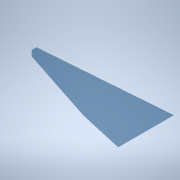
# Autodesk Inventor part: Receivingbeam_OXS200_11728845
Saved by Autodesk Inventor 2021 (Build 250183000, 183)
## iProperties
Created: 2025-06-20
Part Number: Receivingbeam_OXS200_11728845
Material: Generic
Catalog Web Link: www.cadenas.de
Description: ox_receiving_beam-receiving beam
Vendor: BAUMER
Document SubType Name: Modeling
Designer: psAdmin
Manufacturer: BAUMER
Mass: 161.252 g
Surface Area: 402.746 cm^2
Volume: 161.252 cm^3
Density: 1 g/cm^3
Appearance: PSOLRGB-29-191-255
Category: PARTsolutions
Company: BAUMER
Title: Receivingbeam_OXS200_11728845
Author: Cadenas PARTsolutions
Comments: receiving beam
PSOL_IDENT_0: {$CADENAS_DATA/23d-libs/baumer/products/smartvisionsensors/smartprofilesensors/oxmp/oxmp_receiving_b
PSOL_IDENT_1: eam.prj},210 {VTYP=3D},{NB=Receivingbeam_OXS200_11728845},{LINA=Receivingbeam_OXS200_11728845},{NN=o
PSOL_IDENT_2: x_receiving_beam},{DATE=12.06.2025 11:27:17},{GEOMDATE=06.05.2025 06:43:50},{VERSION=},{LINEID=350},
PSOL_IDENT_3: {WBVAR=},{WBNUMERIC=}  {NB=Receivingbeam_OXS200_11728845},{LINA=Receivingbeam_OXS200_11728845},{KT=D
PSOL_IDENT_4: UMMY},{TYPE=Measuring mode (E): Edge, Width/Gap, Intensity Edge, Segment Selector, Caliper X/Z/Dista
PSOL_IDENT_5: nce},{LWL=Red (660 nm)},{MR=100},{TC=OXS200-R10A.E02},{TCX=OXS200},{AN=11728845},{WS=icon_website.pn
PSOL_IDENT_6: g},{EP=eplan_data_standard.png},{MH=Aluminium},{MO=Glass},{WT=270},{PC=IP 65},{LC=2},{ET=18 … 30 VDC
PSOL_IDENT_7: },{AOS=4-20mA, 2-10mA, 0-10V, 0-5V},{SO=2 x Outputs (Push-Pull)},{CONS=typ. 2.4W (100 mA max at 24 V
PSOL_IDENT_8: ) | IEEE 802.3af Power over Ethernet (PoE)},{OT=0 ... + 45 °C},{ALI=< 25 kLux},{CS=CE, UL, PROFINET,
PSOL_IDENT_9: ETHERNET/IP},{EC=t.b.d.},{CTN=t.b.d.},{COO=t.b.d.},{TYPEX=1},{LWLX=1},{B0R=7.500},{H0=3.000},{SDC=1
PSOL_IDENT_10: 50.000},{B1=75.000},{H1=0.650},{B2R=125.000},{H2=0.750},{EH=8.500},{RH=37.300},{RW=12.000},{HX=0.400
PSOL_IDENT_11: },{L2=250.000}
NB: Receivingbeam_OXS200_11728845
NN: ox_receiving_beam
NT: receiving beam
NBSYN: Receivingbeam_$TCX._$AN.
LINA: Receivingbeam_OXS200_11728845
CATALOG: Baumer Group
TYPE: Measuring mode (E): Edge, Width/Gap, Intensity Edge, Segment Selector, Caliper X/Z/Distance
LWL: Red (660 nm)
MR: 100
TC: OXS200-R10A.E02
TCX: OXS200
AN: 11728845
WS: icon_website.png
EP: eplan_data_standard.png
MH: Aluminium
MO: Glass
WT: 270
PC: IP 65
LC: 2
ET: 18 … 30 VDC
AOS: 4-20mA, 2-10mA, 0-10V, 0-5V
SO: 2 x Outputs (Push-Pull)
CONS: typ. 2.4W (100 mA max at 24 V) | IEEE 802.3af Power over Ethernet (PoE)
OT: 0 ... + 45 °C
ALI: < 25 kLux
CS: CE, UL, PROFINET, ETHERNET/IP
EC: t.b.d.
CTN: t.b.d.
COO: t.b.d.
B0R: 7.5
B2R: 125
HX: 0.4
L2: 250
SUPPLIER: BAUMER
ARTICLENO: Receivingbeam_OXS200_11728845
BOMINFO: Receivingbeam_OXS200_11728845
CREATOR: CADENAS GmbH
Autodesk Inventor part; units mm, degrees
sketch "Sketch_4" plane through (0, 0, 0) normal (0, 0, 1) x (1, 0, 0)
  line L0 (-1.9813, 35.0728) -> (-1.9773, 23.1005)
  line L1 (-1.9773, 23.1005) -> (150, 0)
  line L2 (150, 0) -> (250, 0)
  line L3 (250, 0) -> (250, 0.375)
  line L4 (250, 0.375) -> (-1.9813, 35.0728)
  constraints: 10 end point
extrude "Extrusion1" add sketch "Sketch_4" along normal mid plane 129
sketch "Sketch_5" plane through (0, 0, 0) normal (0, 1, 0) x (-1, 0, 0)
  line L0 (5, 131) -> (-260, 131)
  line L1 (-260, 131) -> (-260, -131)
  line L2 (-260, -131) -> (5, -131)
  line L3 (5, -131) -> (5, 131)
  line L4 (2.9262, 5.3387) -> (-250, 62.5)
  line L5 (-250, 62.5) -> (-250, -62.5)
  line L6 (-250, -62.5) -> (2.9262, -5.3387)
  line L7 (2.9262, -5.3387) -> (2.9262, 5.3387)
  constraints: 16 end point
extrude "Extrusion2" cut sketch "Sketch_5" along normal mid plane 91.6
ref_plane "CP1_XY" through (0, 0, 0) normal (0, 0, 1) x (1, 0, 0)
ref_plane "CP1_YZ" through (0, 0, 0) normal (1, 0, 0) x (0, 1, 0)
ref_plane "CP1_ZX" through (0, 0, 0) normal (0, 1, 0) x (0, 0, 1)
body "Solid1"
